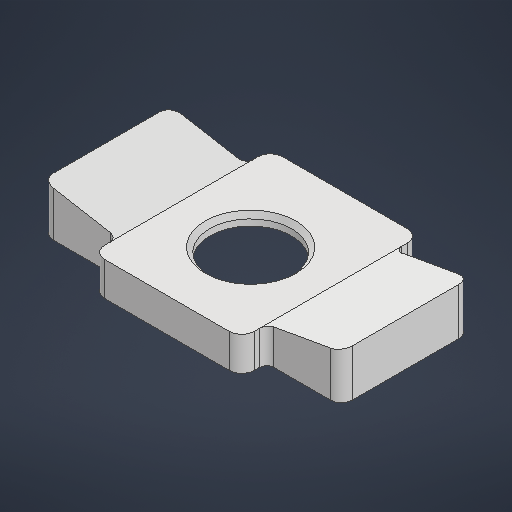
# Autodesk Inventor part: Part1
Saved by Autodesk Inventor 2026 (Build 300175000, 175)
## iProperties
Created: 2025-04-13
Part Number: Part1
Material: Generic
Document SubType Name: Modeling
Designer: ct_vi
Density: 1 g/cm^3
Appearance: Default
Author: ct_vi
Autodesk Inventor part; units mm, degrees
ref_plane "YZ Plane" through (0, 0, 0) normal (1, 0, 0) x (0, 1, 0)
ref_plane "XZ Plane" through (0, 0, 0) normal (0, 1, 0) x (-1, 0, 0)
sketch "Sketch1" plane through (0, 0, 0) normal (0, 1, 0) x (-1, 0, 0)
  circle A0 centre (0, 1.5) radius 11.5
  circle A1 centre (0, 1.5) radius 12.5
  line L0 (19.0144, -21.3297) -> (-18.8688, -21.3297) construction
  line L1 (-18.8688, -21.3297) -> (-18.8688, 21.6448) construction
  line L2 (-18.8688, 21.6448) -> (19.0144, 21.6448) construction
  line L3 (19.0144, 21.6448) -> (19.0144, -21.3297) construction
  line L4 (-2.25, -4) -> (-2.25, -8.7)
  line L5 (-2.25, -8.7) -> (2.25, -8.7)
  line L6 (2.25, -8.7) -> (2.25, -4)
  line L7 (2.25, -4) -> (-2.25, -4)
  line L8 (5.9381, 2.2148) -> (9.8353, 4.4648)
  line L9 (9.8353, 4.4648) -> (7.4853, 8.5352)
  line L10 (7.4853, 8.5352) -> (3.5881, 6.2852)
  line L11 (5.9381, 2.2148) -> (3.5881, 6.2852)
  line L12 (-3.5881, 6.2852) -> (-7.4853, 8.5352)
  line L13 (-7.4853, 8.5352) -> (-9.8353, 4.4648)
  line L14 (-9.8353, 4.4648) -> (-5.9381, 2.2148)
  line L15 (-3.5881, 6.2852) -> (-5.9381, 2.2148)
  circle A2 centre (10.199, -17.6855) radius 1.5
  circle A3 centre (-10.301, 18.0645) radius 1.5
  circle A4 centre (10.199, 18.0645) radius 1.5
  circle A5 centre (-10.301, -17.6855) radius 1.5
  line L16 (10.199, -17.6855) -> (-10.301, -17.6855)
  line L17 (-10.301, -17.6855) -> (-10.301, 18.0645)
  line L18 (-10.301, 18.0645) -> (10.199, 18.0645)
  line L19 (10.199, 18.0645) -> (10.199, -17.6855)
  line L20 (18, -22) -> (-18, -22)
  line L21 (-18, -22) -> (-18, 22)
  line L22 (-18, 22) -> (18, 22)
  line L23 (18, 22) -> (18, -22)
  line L24 (18, -22) -> (-18, 22) construction
  line L25 (-18, -22) -> (18, 22) construction
  line L26 (0, 0) -> (20.5, 0)
  line L27 (0, 0) -> (0, 25)
  line L28 (17.5, -25) -> (-17.5, -25)
  line L29 (-21, -21.5) -> (-21, 21.5)
  line L30 (-17.5, 25) -> (17.5, 25)
  line L31 (21, -25) -> (-21, 25) construction
  line L32 (-21, -25) -> (21, 25) construction
  arc A6 (-17.5, 25) -> (-21, 21.5) centre (-17.5, 21.5) ccw
  arc A7 (-21, -21.5) -> (-17.5, -25) centre (-17.5, -21.5) ccw
  line L33 (17.5, -23) -> (-17.5, -23)
  line L34 (-19, -21.5) -> (-19, 21.5)
  line L35 (-17.5, 23) -> (17.5, 23)
  line L36 (19, 21.5) -> (19, -21.5)
  line L37 (19, -23) -> (-19, 23) construction
  line L38 (-19, -23) -> (19, 23) construction
  arc A8 (-17.5, 23) -> (-19, 21.5) centre (-17.5, 21.5) ccw
  arc A9 (-19, -21.5) -> (-17.5, -23) centre (-17.5, -21.5) ccw
  line L39 (9.2678, 19.2405) -> (9.2678, 16.8886)
  line L40 (9.2678, -16.5095) -> (9.2678, -18.8614)
  line L41 (-9.3698, 19.2405) -> (-9.3698, 16.8886)
  line L42 (-9.3698, -16.5095) -> (-9.3698, -18.8614)
  line L43 (17.5, -24) -> (-17.5, -24)
  line L44 (-20, -21.5) -> (-20, 21.5)
  line L45 (-17.5, 24) -> (17.5, 24)
  line L46 (20, -24) -> (-20, 24) construction
  line L47 (-20, -24) -> (20, 24) construction
  arc A10 (-17.5, 24) -> (-20, 21.5) centre (-17.5, 21.5) ccw
  arc A11 (-20, -21.5) -> (-17.5, -24) centre (-17.5, -21.5) ccw
  line L48 (21, -21.5) -> (21, 21.5)
  line L49 (20, 21.5) -> (20, -21.5)
  arc A12 (17.5, -24) -> (20, -21.5) centre (17.5, -21.5) ccw
  arc A13 (17.5, -25) -> (21, -21.5) centre (17.5, -21.5) ccw
  arc A14 (17.5, -23) -> (19, -21.5) centre (17.5, -21.5) ccw
  arc A15 (21, 21.5) -> (17.5, 25) centre (17.5, 21.5) ccw
  arc A16 (20, 21.5) -> (17.5, 24) centre (17.5, 21.5) ccw
  arc A17 (19, 21.5) -> (17.5, 23) centre (17.5, 21.5) ccw
  line L50 (19, 0) -> (39, 0)
  line L51 (39, 0) -> (39, -15)
  line L52 (39, -15) -> (19, -15)
  line L53 (19, -15) -> (19, 15)
  line L54 (19, 15) -> (39, 15)
  line L55 (39, 15) -> (39, -15)
  line L56 (39, 16) -> (19, 16)
  line L57 (19, 16) -> (19, -16)
  line L58 (39, 0) -> (42, 0)
  line L59 (39, 0) -> (40, 0)
  line L60 (40, 0) -> (40, -16)
  line L61 (39, -16) -> (19, -16)
  line L62 (19, -16) -> (19, 16)
  line L63 (40, 15) -> (40, -15)
  line L64 (40, 0) -> (41, 0)
  line L65 (41, 0) -> (41, -17)
  line L66 (39, -17) -> (20, -17)
  line L67 (20, -17) -> (20, 17)
  line L68 (20, 17) -> (39, 17)
  line L69 (41, 15) -> (41, -15)
  line L70 (41, 0) -> (42, 0)
  line L71 (42, 0) -> (42, -15)
  line L72 (39, -18) -> (21, -18)
  line L73 (21, -18) -> (21, 18)
  line L74 (21, 18) -> (39, 18)
  line L75 (42, 15) -> (42, -18)
  arc A18 (39, -16) -> (40, -15) centre (39, -15) ccw
  arc A19 (40, 15) -> (39, 16) centre (39, 15) ccw
  arc A20 (39, -17) -> (41, -15) centre (39, -15) ccw
  arc A21 (41, 15) -> (39, 17) centre (39, 15) ccw
  arc A22 (39, -18) -> (42, -15) centre (39, -15) ccw
  arc A23 (42, 15) -> (39, 18) centre (39, 15) ccw
  line L76 (19, -15) -> (21.5, -15)
  line L77 (21.5, -15) -> (21.5, 16)
  line L78 (21.5, 16) -> (19, 16)
  line L79 (19, 16) -> (19, -15)
  line L80 (-19, 0) -> (-39, 0)
  line L81 (-39, 0) -> (-39, -15)
  line L82 (-39, -15) -> (-19, -15)
  line L83 (-19, -15) -> (-19, 15)
  line L84 (-19, 15) -> (-39, 15)
  line L85 (-39, 15) -> (-39, -15)
  line L86 (-39, 0) -> (-40, 0)
  line L87 (-19, -16) -> (-19, 16)
  line L88 (-40, 0) -> (-41, 0)
  line L89 (-41, 0) -> (-42, 0)
  line L90 (-42, 0) -> (-42, -15)
  line L91 (-21, -18) -> (-21, 19)
  line L92 (-20, -17) -> (-20, 17)
  line L93 (-41, 0) -> (-41, -15)
  line L94 (-41, 0) -> (-26, 0) construction
  line L95 (-20, -17) -> (-20, 17)
  line L96 (-40, 0) -> (-40, -16)
  line L97 (-40, 0) -> (-24, 0) construction
  line L98 (-39, -16) -> (-19, -16)
  line L99 (-19, -16) -> (-19, 16)
  line L100 (-19, 16) -> (-39, 16)
  line L101 (-40, 15) -> (-40, -15)
  arc A24 (-40, -15) -> (-39, -16) centre (-39, -15) ccw
  arc A25 (-39, 16) -> (-40, 15) centre (-39, 15) ccw
  line L102 (-39, -17) -> (-20, -17)
  line L103 (-41, 0) -> (-41, 15)
  line L104 (-39, 17) -> (-20, 17)
  arc A26 (-41, -15) -> (-39, -17) centre (-39, -15) ccw
  arc A27 (-39, 17) -> (-41, 15) centre (-39, 15) ccw
  line L105 (-39, -18) -> (-21, -18)
  line L106 (-42, 0) -> (-42, 15)
  line L107 (-39, 18) -> (-21, 18)
  arc A28 (-42, -15) -> (-39, -18) centre (-39, -15) ccw
  arc A29 (-39, 18) -> (-42, 15) centre (-39, 15) ccw
  line L108 (-19, 16) -> (-21.5, 16)
  line L109 (-21.5, 16) -> (-21.5, -16)
  line L110 (-21.5, -16) -> (-19, -16)
  line L111 (-19, -16) -> (-19, 16)
  point P0 (21, -22)
  point P1 (21, 22)
  point P2 (19, 24)
  point P3 (19, -24)
  point P4 (40, 16)
  point P5 (42, 18)
  point P6 (20, -15)
  point P7 (21.5, 15)
  point P8 (20, 15)
  point P9 (-42, -18)
  point P10 (-41, -17)
  point P11 (-40, 16)
  point P12 (-41, 17)
  point P13 (-42, 18)
  point P14 (-20, 17)
  point P15 (41, -15)
  point P16 (-20, -16)
  point P17 (-21, -17)
  point P18 (-21, -16)
  dimension "d33" = 4.7
  dimension "d34" = 4.5
  dimension "d36" = 4.5
  dimension "d37" = 4.7
  dimension "d38" = 3
  dimension "d46" = 3
  dimension "d47" = 3
  dimension "d48" = 3
  dimension "d166" = 50
  dimension "d193" = 48
  dimension "d210" = 46
  dimension "d211" = 1.5
  dimension "d212" = 2.5
  dimension "d216" = 3.5
  dimension "d217" = 44
  dimension "d245" = 2.5
  dimension "d246" = 3.5
  dimension "d247" = 1.5
  dimension "d248" = 3.5
  dimension "d249" = 2.5
  dimension "d250" = 1.5
  dimension "d261" = 20
  dimension "d262" = 15
  dimension "d264" = 30
  dimension "d304" = 1
  dimension "d305" = 16
  dimension "d306" = 21
  dimension "d307" = 1
  dimension "d308" = 17
  dimension "d310" = 34
  dimension "d311" = 1
  dimension "d312" = 18
  dimension "d313" = 21
  dimension "d314" = 36
  dimension "d315" = 1
  dimension "d316" = 2
  dimension "d317" = 3
  dimension "d318" = 2.5
  dimension "d328" = 1
  dimension "d330" = 1
  dimension "d332" = 1
  dimension "d333" = 18
  dimension "d338" = 17
  dimension "d343" = 16
  dimension "d345" = 21
  dimension "d346" = 1
  dimension "d347" = 17
  dimension "d348" = 2
  dimension "d349" = 18
  dimension "d350" = 3
  dimension "d366" = 2.5
  constraints: 216 end point, 59 point on line, 56 point on circle, 48 tangent, 30 centre point, 30 perpendicular, 25 parallel, 24 horizontal, 10 midpoint, 6 equal radius, 5 vertical, 2 other
  measures "d33" distance of L4.start L4.end
  measures "d34" distance of L4.end L5.end
  measures "d36" distance of L8.start L8.end
  measures "d37" distance of L8.end L9.end
  measures "d38" diameter of A2
  measures "d46" diameter of A3
  measures "d47" diameter of A4
  measures "d48" diameter of A5
  measures "d166" distance of L32.start L31.end
  measures "d193" distance of L47.start L46.end
  measures "d210" distance between parallel lines of L35 L33
  measures "d211" radius of A9
  measures "d212" radius of A11
  measures "d216" radius of A7
  measures "d217" distance between parallel lines of L22 L20
  measures "d245" radius of A12
  measures "d246" radius of A13
  measures "d247" radius of A14
  measures "d248" radius of A15
  measures "d249" radius of A16
  measures "d250" radius of A17
  measures "d261" distance of L50.start L50.end
  measures "d262" distance of L50.end L51.end
  measures "d264" distance of L52.end L53.end
  measures "d304" distance of L50.end L59.end
  measures "d305" distance of L59.end L60.end
  measures "d306" distance of L56.end point (40, 16)
  measures "d307" distance of L59.end L64.end
  measures "d308" distance of L64.end L65.end
  measures "d310" distance of L66.end L67.end
  measures "d311" distance of L64.end L58.end
  measures "d312" distance of L58.end L75.end
  measures "d313" distance of L73.end point (42, 18)
  measures "d314" distance of L72.end L73.end
  measures "d315" radius of A18
  measures "d316" radius of A20
  measures "d317" radius of A22
  measures "d318" distance of L78.end L77.end
  measures "d328" distance of L80.end L86.end
  measures "d330" distance of L86.end L88.end
  measures "d332" distance of L88.end L89.end
  measures "d333" distance of L89.end point (-42, -18)
  measures "d338" distance of L88.end point (-41, -17)
  measures "d343" distance of L86.end L96.end
  measures "d345" distance of point (-40, 16) L87.end
  measures "d346" radius of A24
  measures "d347" distance of L88.end point (-41, 17)
  measures "d348" radius of A26
  measures "d349" distance of L89.end point (-42, 18)
  measures "d350" radius of A28
  measures "d366" distance of L110.end L109.end
extrude "Extrusion1" add sketch "Sketch1" against normal blind 2.5 contours A0 L19 A1 L26 | A0 L27 A1 L19 | L26 A1 L19 A0 | A0 L17 A1 L27 | L19 A1 L17 A0 | A0 L17 A1
extrude "Extrusion4" add sketch "Sketch1" against normal blind 5 contours L19 L18 L39 A4 | A4 L39 L18 L19 | A4 L18 L39 | L19 L16 L40 A2 | A2 L40 L16 L19 | L17 L18 L41 A3 | A3 L41 L18 L17 | L18 L41 A3 | A3 L41 L18 | A4 L39 L18 | L17 L16 L42 A5 | A5 L42 L16 L17 | L40 L16 A2 | A5 L16 L42 | L42 L16 A5 | A2 L16 L40
extrude "Extrusion11" add sketch "Sketch1" against normal blind 1 contours L19 A4 L18 L27 L22 L23 L26 A1 | A1 L27 L18 A4 L19 | L26 L23 L20 L21 L22 L27 L18 A3 L17 A1 A5 L16 A2 L19 | A1 L17 A3 L18 L27 | L19 A2 L16 A5 L17 A1
extrude "Extrusion13" add sketch "Sketch1" along normal blind 0.5 contours A0 L19 A1 L26 | A0 L27 A1 L19 | L26 A1 L19 A0 | A0 L17 A1 L27 | L19 A4 L18 L27 L22 L23 L26 A1 | A1 L27 L18 A4 L19 | L19 A1 L17 A0 | L26 L23 L20 L21 L22 L27 L18 A3 L17 A1 A5 L16 A2 L19 | A0 L17 A1 | A1 L17 A3 L18 L27 | L19 L18 L39 A4 | A4 L39 L18 L19 | L19 A2 L16 A5 L17 A1 | L26 L36 A14 L33 A9 L34 A8 L35 L27 L22 L21 L20 L23 | L23 L22 L27 L35 A17 L36 L26 | A4 L18 L39 | L19 L16 L40 A2 | A2 L40 L16 L19 | L17 L18 L41 A3 | A3 L41 L18 L17 | L18 L41 A3 | A3 L41 L18 | A4 L39 L18 | L17 L16 L42 A5 | A5 L42 L16 L17 | L40 L16 A2 | A5 L16 L42 | L42 L16 A5 | A2 L16 L40
extrude "Extrusion15" add sketch "Sketch1" against normal blind 1 contours L26 L36 A14 L33 A9 L34 A8 L35 L27 L22 L21 L20 L23 | L23 L22 L27 L35 A17 L36 L26
extrude "Extrusion16" cut sketch "Sketch1" against normal through all contours A4 L18 L39 | L18 L41 A3 | A3 L41 L18 | A4 L39 L18 | L40 L16 A2 | A5 L16 L42 | L42 L16 A5 | A2 L16 L40
chamfer "Chamfer2" distance 1.25 angle 45 1 edges at (11.5, 0.5, 1.5)
chamfer "Chamfer3" distance 0.5 angle 45 1 edges at (12.5, -1, 1.5)
extrude "Extrusion22" add sketch "Sketch1" along normal blind 0.5 contours L49 L54 L48 L50 L26 | L26 L50 L48 L52 L49 | L49 L56 L48 L54 | L52 L48 L61 L49 | L45 A10 L44 L104 L29 A6 L30 L27 | L27 L30 A15 L48 L68 L49 A16 L45 | L50 L77 L52 L48 | L48 L54 L77 L50 | L49 L68 L48 L56 | L48 L56 L77 L54 | L61 L48 L66 L49 | L52 L51 L58 L60 A18 L61 L48 | L77 L54 L55 L50 | L50 L51 L52 L77 | L48 L68 A21 L69 L58 L63 A19 L56 | L77 L56 A19 L63 L58 L55 L54 | L66 L48 A13 L28 A7 L29 L102 L44 A11 L43 A12 L49 | L61 A18 L60 L58 L65 A20 L66 L48 | L48 L74 A23 L75 L58 L69 A21 L68 | L66 A20 L65 L58 L71 A22 L72 L48 | L44 L100 L29 L104 | L44 L84 L29 L100 | L44 L80 L29 L84 | L44 L82 L29 L80 | L98 L29 L82 L44 | L44 L102 L29 L98
extrude "Extrusion23" add sketch "Sketch1" along normal blind 0.5 contours L36 L54 L49 L26 | L26 L49 L52 L36 | L36 L56 L49 L54 | L52 L49 L61 L36 | L35 A8 L34 L100 L44 A10 L45 L27 | L27 L45 A16 L49 L56 L36 A17 L35 | L61 L49 A12 L43 A11 L44 L98 L34 A9 L33 A14 L36 | L34 L84 L44 L100 | L34 L80 L44 L84 | L34 L82 L44 L80 | L98 L44 L82 L34
extrude "Extrusion24" add sketch "Sketch1" against normal blind 2.5 contours L36 L54 L49 L26 | L26 L49 L52 L36 | L49 L54 L48 L50 L26 | L26 L50 L48 L52 L49 | L50 L77 L52 L48 | L48 L54 L77 L50
extrude "Extrusion25" add sketch "Sketch1" along normal blind 0.5 contours L104 A27 L103 L89 L106 A29 L107 L29 | L29 L100 A25 L101 L88 L103 A27 L104 | L29 L84 L109 L100 | L29 L80 L109 L84 | L109 L84 L85 L86 L101 A25 L100 | L29 L82 L109 L80 | L109 L80 L85 L84 | L98 L109 L82 L29 | L29 L102 A26 L93 L88 L96 A24 L98 | L93 A26 L102 L29 L105 A28 L90 L89 | L109 L82 L81 L80 | L98 A24 L96 L86 L81 L82 L109
sketch "Sketch4" plane through (21, 0, 18) normal (0, 0, 1) x (1, 0, 0)
  line L0 (0, 0) -> (18, 0) projected
  line L1 (0, 0) -> (0, 0.5) projected
  line L2 (0, 0) -> (0, 0.5)
  line L3 (0, 0.5) -> (21, 0.5)
  line L4 (21, 0.5) -> (21, 4.2029)
  line L5 (21, 4.2029) -> (0, 0.5)
  point P0 (-21, 0)
  dimension "d353" = 21
  dimension "d354" = 90
  dimension "d355" = 10
  constraints: 8 end point, 1 perpendicular, 1 vertical
  measures "d353" distance of L1.end L3.end
  measures "d354" angle of L4 L3
  measures "d355" angle of L3 L5
extrude "Extrusion26" add sketch "Sketch4" against normal blind 36
fillet "Fillet6" radius 3 2 edges at (42, 2.3514, 18) (42, 2.3514, -18)
sketch "Sketch5" plane through (0, 0, 0) normal (0, -1, 0) x (1, 0, 0)
  point P0 (0, 0)
ref_plane "Work Plane2" through (19, 0, 0) normal (0, 0, -1) x (1, 0, 0)
sketch "Sketch6" plane through (19, 0, 0) normal (0, 0, -1) x (1, 0, 0)
  line L0 (20, 0) -> (23, 0) projected
  line L1 (23, 0) -> (21, 0)
  line L2 (21, 0) -> (21, -3.3502)
  line L3 (2, -0.5) -> (2, 0) projected
  line L4 (21, -3.3502) -> (2, 0)
  line L5 (2, 0) -> (21, 0)
  line L6 (-38, 0) -> (-40, 0)
  line L7 (-40, 0) -> (-59, 0)
  line L8 (-59, 0) -> (-59, -3.3502)
  line L9 (-59, -3.3502) -> (-40, 0)
  point P0 (-19, 0)
  dimension "d361" = 2
  dimension "d362" = 10
  dimension "d380" = 2
  dimension "d381" = 19
  dimension "d382" = 10
  constraints: 16 end point, 2 horizontal, 2 perpendicular, 2 point on line
  measures "d361" distance of L0.end L1.end
  measures "d362" angle of L5 L4
  measures "d380" distance of L6.start L6.end
  measures "d381" distance of L6.end L7.end
  measures "d382" angle of L7 L9
extrude "Extrusion27" cut sketch "Sketch6" along normal mid plane 32 contours L0 L2 L4 L5
fillet "Fillet7" radius 1 2 edges at (40, 1.6751, -16) (40, 1.6751, 16)
extrude "Extrusion28" add sketch "Sketch1" against normal blind 2.5 contours L34 L84 L44 L100 | L34 L80 L44 L84 | L44 L84 L29 L100 | L34 L82 L44 L80 | L44 L80 L29 L84 | L29 L84 L109 L100 | L98 L44 L82 L34 | L44 L82 L29 L80 | L29 L80 L109 L84 | L98 L29 L82 L44 | L29 L82 L109 L80 | L98 L109 L82 L29
sketch "Sketch7" plane through (-39, 0, -18) normal (0, 0, -1) x (-1, 0, 0)
  line L0 (-18, 0.5) -> (0, 0.5) projected
  line L1 (3, 0.5) -> (0, 0.5) projected
  line L2 (-18, 0.5) -> (3, 0.5)
  line L3 (-18, 0.5) -> (3, 0.5) construction
  line L4 (3, 0.5) -> (3, 4.2029)
  line L5 (3, 4.2029) -> (-18, 0.5)
  point P0 (-39, 0)
  point P1 (-16.25, 0.5)
  point P2 (-16.25, 0.5)
  dimension "d376" = 0
  dimension "d377" = 10
  constraints: 8 end point, 2 horizontal, 1 collinear, 1 perpendicular
  measures "d376" distance between parallel lines of L2 L3
  measures "d377" angle of L5 L0
extrude "Extrusion31" add sketch "Sketch7" against normal blind 36
extrude "Extrusion32" cut sketch "Sketch6" along normal mid plane 32 contours L9 L8 L7
fillet "Fillet10" radius 1 2 edges at (-40, 1.6751, -16) (-40, 1.6751, 16)
fillet "Fillet11" radius 3 2 edges at (-42, 2.3514, -18) (-42, 2.3514, 18)
extrude "Outer_Shell" add sketch "Sketch1" against normal blind 9 contours L45 A10 L44 L104 L29 A6 L30 L27 | L27 L30 A15 L48 L68 L49 A16 L45 | L66 L48 A13 L28 A7 L29 L102 L44 A11 L43 A12 L49 | L48 L74 A23 L75 L58 L69 A21 L68 | L66 A20 L65 L58 L71 A22 L72 L48 | L104 A27 L103 L89 L106 A29 L107 L29 | L93 A26 L102 L29 L105 A28 L90 L89
extrude "Extrusion34" add sketch "Sketch1" against normal blind 8 contours L35 A8 L34 L100 L44 A10 L45 L27 | L27 L45 A16 L49 L56 L36 A17 L35 | L61 L49 A12 L43 A11 L44 L98 L34 A9 L33 A14 L36 | L49 L68 L48 L56 | L61 L48 L66 L49 | L48 L68 A21 L69 L58 L63 A19 L56 | L61 A18 L60 L58 L65 A20 L66 L48 | L44 L100 L29 L104 | L29 L100 A25 L101 L88 L103 A27 L104 | L44 L102 L29 L98 | L29 L102 A26 L93 L88 L96 A24 L98
fillet "Fillet12" radius 2 4 edges at (21, -4.25, -18) (-21, -4.25, -18) (21, -4.25, 18) (-21, -4.25, 18)
body "Solid1"
